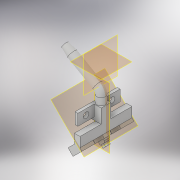
# Autodesk Inventor part: LickSensorMount_H
Saved by Autodesk Inventor 2020 (Build 240168000, 168)
## iProperties
Created: 2019-07-29
Part Number: LickSensorMount_H
Material: 일반
Document SubType Name: Modeling
Designer: Jeong Ji Hoon
Density: 1 g/cm^3
Appearance: 기본값
Author: Jeong Ji Hoon
## iProperties of the stored document _3D 인쇄.ipt
Created: 2020-01-15
Part Number: _3D 인쇄
Material: 일반
Document SubType Name: Modeling
Designer: Knowblesse
Density: 1 g/cm^3
Appearance: 기본값
Author: Knowblesse
Autodesk Inventor part; units mm, degrees
ref_plane "YZ Plane" through (0, 0, 0) normal (1, 0, 0) x (0, 1, 0)
ref_plane "XZ Plane" through (0, 0, 0) normal (0, 1, 0) x (-1, 0, 0)
ref_plane "XY Plane" through (0, 0, 0) normal (0, 0, 1) x (1, 0, 0)
sketch "스케치1" plane through (0, 0, 0) normal (0, 1, 0) x (-1, 0, 0)
  line L0 (0, 0) -> (7, 0)
  line L1 (7, 0) -> (7, -7)
  line L2 (7, -7) -> (0, -7)
  line L3 (0, -7) -> (0, 0)
  dimension "d0" = 7
  dimension "d1" = 7
  constraints: 8 end point, 2 parallel, 1 horizontal, 1 perpendicular
  measures "d0" distance of L1.end L2.end
  measures "d1" distance of L0.end L1.end
extrude "돌출1" add sketch "스케치1" along normal blind 10
sketch "스케치2" plane through (0, 10, 0) normal (0, 1, 0) x (1, 0, 0)
  line L0 (-7, 0) -> (0, 0) projected
  line L1 (0, 0) -> (0, 7) projected
  line L2 (0, 7) -> (-7, 7) projected
  line L3 (-7, 7) -> (-7, 0) projected
  circle A0 centre (-3.5, 3.5) radius 3
  line L4 (-7, 3.5) -> (0, 3.5) construction
  line L5 (-3.5, 7) -> (-3.5, 0) construction
  point P0 (-3.5, 3.5)
  dimension "d4" = 6
  constraints: 5 midpoint, 4 end point, 1 centre point, 1 coincident
  measures "d4" diameter of A0
extrude "돌출2" add sketch "스케치2" along normal blind 25 contours A0
ref_plane "작업 평면1" through (-3.5, 0, 0) normal (1, 0, 0) x (0, 0, -1)
sketch "스케치5" plane through (0, 0, 0) normal (1, 0, 0) x (0, 0, -1)
  line L0 (7, 0) -> (0, 0) projected
  line L1 (-15, -7) -> (22, -7)
  line L2 (22, -7) -> (22, 0)
  line L3 (22, 0) -> (-15, 0)
  line L4 (-15, 0) -> (-15, -7)
  point P0 (3.5, 0)
  dimension "d16" = 37
  dimension "d17" = 7
  constraints: 8 end point, 2 midpoint, 2 parallel, 1 horizontal, 1 perpendicular
  measures "d16" distance of L1.start L1.end
  measures "d17" distance of L3.end L1.start
extrude "돌출4" add sketch "스케치5" against normal blind 4
sketch "스케치6" plane through (0, 0, 0) normal (0, -1, 0) x (1, 0, 0)
  circle A0 centre (-3.5, -3.5) radius 2.5
  circle A1 centre (-3.5, -3.5) radius 3.5 projected
  dimension "d20" = 5
  constraints: 2 coincident, 1 centre point
  measures "d20" diameter of A0
extrude "돌출5" add sketch "스케치6" along normal blind 11 contours A0
ref_plane "작업 평면2" through (0, -7, 0) normal (0.7071068, 0.7071068, 0) x (0, 0, 1)
sketch "스케치7" plane through (0, -7, 0) normal (0.7071068, 0.7071068, 0) x (0, 0, 1)
  line L0 (-7, -4.9497) -> (-7, -12.0208) projected
  line L1 (0, -12.0208) -> (-7, -12.0208) projected
  line L2 (0, -4.9497) -> (0, -12.0208) projected
  line L3 (0, -4.9497) -> (15, -4.9497) projected
  line L4 (15, -4.9497) -> (15, 0) projected
  line L5 (15, 0) -> (-22, 0) projected
  line L6 (-22, 0) -> (-22, -4.9497) projected
  line L7 (-22, -4.9497) -> (-7, -4.9497) projected
  line L8 (-22, 2) -> (15, 2)
  line L9 (15, 2) -> (15, -3)
  line L10 (15, -3) -> (-22, -3)
  line L11 (-22, -3) -> (-22, 2)
  line L12 (15, -4.9497) -> (15, 0) projected
  dimension "d24" = 5
  dimension "d25" = 2
  constraints: 8 end point, 2 collinear, 2 parallel, 1 horizontal, 1 perpendicular
  measures "d24" distance of L8.end L9.end
  measures "d25" distance between parallel lines of L8 L5
extrude "돌출6" add sketch "스케치7" against normal blind 9 contours L6 L5 L4 L10 | L11 L8 L9 L5
sketch "스케치8" plane through (1.4142, -8.4142, 15) normal (0.7071068, -0.7071068, 0) x (-0.7071068, -0.7071068, 0)
  line L0 (0, 37) -> (0, 0) projected
  line L1 (0, 0) -> (9, 0) projected
  line L2 (9, 37) -> (9, 0) projected
  line L3 (0, 37) -> (9, 37) projected
  line L4 (0.9, 2.5) -> (7.2, 2.5)
  line L5 (7.2, 2.5) -> (7.2, 7.3)
  line L6 (7.2, 7.3) -> (0.9, 7.3)
  line L7 (0.9, 7.3) -> (0.9, 2.5)
  line L8 (0.9, 29.7) -> (7.2, 29.7)
  line L9 (7.2, 29.7) -> (7.2, 34.5)
  line L10 (7.2, 34.5) -> (0.9, 34.5)
  line L11 (0.9, 34.5) -> (0.9, 29.7)
  line L12 (9, 9.3) -> (0, 9.3)
  line L13 (9, 27.7) -> (0, 27.7)
  line L14 (9, 15.8) -> (0, 15.8)
  line L15 (9, 21.2) -> (0, 21.2)
  point P0 (-4.9497, 15)
  dimension "d28" = 6.3
  dimension "d29" = 4.8
  dimension "d31" = 2.5
  dimension "d32" = 1.8
  dimension "d33" = 2.5
  dimension "d34" = 2
  dimension "d35" = 2
  dimension "d36" = 6.5
  dimension "d37" = 6.5
  constraints: 24 end point, 10 point on line, 5 parallel, 5 perpendicular, 2 horizontal, 1 collinear
  measures "d28" distance of L5.end L6.end
  measures "d29" distance of L4.end L5.end
  measures "d31" distance between parallel lines of L1 L4
  measures "d32" distance between parallel lines of L2 L5
  measures "d33" distance between parallel lines of L3 L10
  measures "d34" distance between parallel lines of L6 L12
  measures "d35" distance between parallel lines of L8 L13
  measures "d36" distance between parallel lines of L12 L14
  measures "d37" distance between parallel lines of L13 L15
extrude "돌출7" cut sketch "스케치8" against normal through all contours L13 L2 L15 L0 | L14 L2 L12 L0 | L7 L6 L5 L4 | L11 L10 L9 L8
sketch "스케치9" plane through (1.4142, -8.4142, -0.8) normal (0.7071068, -0.7071068, 0) x (-0.7071068, -0.7071068, 0)
  line L0 (9, 5.4) -> (9, 0) projected
  line L1 (0, 5.4) -> (0, 0) projected
  line L2 (2, 0.7) -> (7, 0.7)
  line L3 (7, 0.7) -> (7, 4.7)
  line L4 (7, 4.7) -> (2, 4.7)
  line L5 (2, 4.7) -> (2, 0.7)
  line L6 (9, 2.7) -> (0, 2.7) construction
  point P0 (-4.9497, -0.8)
  point P1 (2, 2.7)
  dimension "d40" = 4
  dimension "d41" = 5
  dimension "d42" = 2
  constraints: 10 end point, 3 midpoint, 2 parallel, 1 horizontal, 1 perpendicular, 1 point on line
  measures "d40" distance of L2.end L3.end
  measures "d41" distance of L3.end L4.end
  measures "d42" distance between parallel lines of L3 L0
extrude "돌출8" add sketch "스케치9" along normal blind 2
sketch "스케치10" plane through (2.8284, -9.8284, -0.8) normal (0.7071068, -0.7071068, 0) x (0, 0, -1)
  line L0 (0.7, -2) -> (0.7, -7) projected
  line L1 (0.7, -7) -> (4.7, -7) projected
  line L2 (4.7, -7) -> (4.7, -2) projected
  line L3 (0.95, -4) -> (4.45, -4)
  line L4 (4.45, -4) -> (4.45, -6.5)
  line L5 (4.45, -6.5) -> (0.95, -6.5)
  line L6 (0.95, -6.5) -> (0.95, -4)
  point P0 (-0.8, 4.9497)
  dimension "d45" = 3.5
  dimension "d46" = 2.5
  dimension "d47" = 0.5
  dimension "d48" = 0.25
  dimension "d49" = 0.25
  constraints: 8 end point, 2 parallel, 1 horizontal, 1 perpendicular
  measures "d45" distance of L4.end L5.end
  measures "d46" distance of L3.end L4.end
  measures "d47" distance between parallel lines of L5 L1
  measures "d48" distance between parallel lines of L0 L6
  measures "d49" distance between parallel lines of L2 L4
extrude "돌출9" add sketch "스케치10" along normal blind 2
sketch "스케치11" plane through (4.2426, -11.2426, -0.8) normal (0.7071068, -0.7071068, 0) x (-0.7071068, -0.7071068, 0)
  line L0 (4, 4.45) -> (4, 0.95) projected
  line L1 (4, 0.95) -> (6.5, 0.95) projected
  line L2 (6.5, 0.95) -> (6.5, 4.45) projected
  line L3 (6.5, 4.45) -> (4, 4.45) projected
  line L4 (4.5, 1.45) -> (4.5, 3.95)
  line L5 (4.5, 3.95) -> (6, 3.95)
  line L6 (6, 3.95) -> (6, 1.45)
  line L7 (6, 1.45) -> (4.5, 1.45)
  point P0 (-4.9497, -0.8)
  dimension "d52" = 0.5
  constraints: 8 end point, 3 other
  measures "d52" distance between parallel lines of L0 L4
extrude "돌출10" cut sketch "스케치11" against normal blind 8 contours L4 L5 L6 L7
ref_plane "작업 평면3" through (-7, 10, -3.5) normal (0, 0, 1) x (1, 0, 0)
chamfer "모따기1" distance 1 angle 45 1 edges at (1.4142, -11.2426, -3.5)
sketch "스케치13" plane through (-4, -6.7574, 5.7) normal (0, 0, -1) x (-1, 0, 0)
  line L0 (0, 3.7574) -> (0, 0) projected
  line L1 (0, 0) -> (4.4853, -4.4853) projected
  line L2 (4.4853, -4.4853) -> (0.9497, -8.0208) projected
  line L3 (0.9497, -8.0208) -> (-5.4142, -1.6569) projected
  line L4 (-5.4142, -1.6569) -> (-4, -0.2426) projected
  line L5 (0, 3.7574) -> (-4, -0.2426) projected
  line L6 (0, 6.7574) -> (0, 3.7574) projected
  line L7 (-4, 6.7574) -> (0, 6.7574) projected
  line L8 (-4, -0.2426) -> (-4, 6.7574) projected
  line L9 (0, 0) -> (4.4853, -4.4853) projected
  line L10 (0, 3.7574) -> (0, 0) projected
  line L11 (0, 6.7574) -> (4.4853, -4.4853)
  point P0 (-1.1716, 1.1716)
  point P1 (0, 1.1716)
  constraints: 2 end point
extrude "돌출12" add sketch "스케치13" against normal up to surface (2 mm away) contours L6 L11 L1 L0
sketch "스케치14" plane through (-4, -6.7574, -12.7) normal (0, 0, 1) x (1, 0, 0)
  line L0 (-0.9497, -8.0208) -> (-4.4853, -4.4853) projected
  line L1 (-4.4853, -4.4853) -> (0, 0) projected
  line L2 (0, 0) -> (0, 3.7574) projected
  line L3 (4, -0.2426) -> (0, 3.7574) projected
  line L4 (4, -0.2426) -> (5.4142, -1.6569) projected
  line L5 (5.4142, -1.6569) -> (-0.9497, -8.0208) projected
  line L6 (0, 3.7574) -> (0, 6.7574) projected
  line L7 (0, 6.7574) -> (4, 6.7574) projected
  line L8 (4, 6.7574) -> (4, -0.2426) projected
  line L9 (0, 6.7574) -> (-4.4853, -4.4853)
  constraints: 2 end point
extrude "돌출13" add sketch "스케치14" against normal up to surface (2 mm away) contours L9 L6 L2 L1
ref_plane "작업 평면4" through (-3.5, 35, -3.5) normal (0, 1, 0) x (1, 0, 0)
sketch "스케치15" plane through (-3.5, 35, -3.5) normal (0, 1, 0) x (1, 0, 0)
  circle A0 centre (0, 0) radius 3.5 projected
  circle A1 centre (0, 0) radius 0.75
  point P0 (3.5, -3.5)
  dimension "d68" = 1.5
  constraints: 1 centre point, 1 coincident
  measures "d68" diameter of A1
extrude "돌출14" cut sketch "스케치15" against normal up to next contours A1
sketch "스케치16" plane through (-7, 0, 0) normal (-1, 0, 0) x (0, 0, 1)
  line L0 (0, 0) -> (-7, 0) projected
  line L1 (0, 0) -> (0, 10) projected
  line L2 (-7, 10) -> (0, 10) projected
  line L3 (-7, 0) -> (-7, 10) projected
  line L4 (11.5, 10) -> (-18.5, 10)
  line L5 (-18.5, 10) -> (-18.5, 2)
  line L6 (-18.5, 2) -> (11.5, 2)
  line L7 (11.5, 2) -> (11.5, 10)
  point P0 (-3.5, 10)
  dimension "d71" = 30
  dimension "d82" = 8
  constraints: 8 end point, 2 midpoint, 2 parallel, 1 collinear, 1 horizontal, 1 perpendicular
  measures "d71" distance of L5.end L6.end
  measures "d82" distance of L6.end L4.start
extrude "돌출15" add sketch "스케치16" against normal blind 2 contours L1 L4 L7 L6 | L6 L5 L4 L3
sketch "스케치17" plane through (-5, 0, 0) normal (1, 0, 0) x (0, 0, -1)
  line L0 (18.5, 2) -> (18.5, 10) projected
  line L1 (0, 0) -> (7, 0) projected
  line L2 (-11.5, 2) -> (-11.5, 10) projected
  line L3 (-11.5, 10) -> (18.5, 10) projected
  line L4 (18.5, 10) -> (18.5, 2) projected
  circle A0 centre (-5.75, 6) radius 2
  circle A1 centre (12.75, 6) radius 2
  line L5 (0, 0) -> (0, 2) projected
  line L6 (0, 2) -> (-11.5, 2) projected
  line L7 (18.5, 2) -> (7, 2) projected
  line L8 (7, 0) -> (7, 2) projected
  dimension "d74" = 4
  dimension "d75" = 4
  dimension "d76" = 5.75
  dimension "d77" = 5.75
  dimension "d81" = 4
  constraints: 2 centre point, 1 horizontal alignment
  measures "d74" diameter of A0
  measures "d75" diameter of A1
  measures "d76" distance from line of L0 A1.centre
  measures "d77" distance from line of L2 A0.centre
  measures "d81" distance from line of L3 A0.centre
extrude "돌출16" cut sketch "스케치17" against normal through all contours A0 | A1
sketch "스케치22" plane through (-3.5, 0, 0) normal (1, 0, 0) x (0, 0, -1)
  line L0 (6.5, 35) -> (0.5, 35) projected
  line L1 (0.5, 10) -> (6.5, 10) projected
  line L2 (0.5, 10) -> (0.5, 35) projected
  line L3 (2.75, 35) -> (4.25, 35) projected
  line L4 (3.5, 35) -> (3.5, 40)
  line L5 (6.5, 35) -> (0.5, 35) projected
  line L6 (0.5, 35) -> (0.5, 41)
  line L7 (0.5, 41) -> (1.3, 47)
  line L8 (1.3, 47) -> (2.1, 47)
  line L9 (2.1, 47) -> (2.1, 37)
  line L10 (2.1, 37) -> (2.75, 35)
  point P0 (0, 0)
  dimension "d113" = 5
  dimension "d114" = 10
  dimension "d115" = 2
  dimension "d116" = 0.8
  dimension "d117" = 6
  dimension "d118" = 2.8
  constraints: 12 end point, 2 perpendicular, 2 vertical, 1 midpoint
  measures "d113" distance of L4.start L4.end
  measures "d114" distance of L8.end L9.end
  measures "d115" distance from line of L9.end L0
  measures "d116" distance of L7.end L8.end
  measures "d117" vertical distance of L7.end L6.end
  measures "d118" diameter of L9 L4
revolve "회전4" add sketch "스케치22" angle 360 about axis through (-3.5, 35, -3.5) along (0, 1, 0)
sketch "스케치20" plane through (-3.5, 0, 0) normal (1, 0, 0) x (0, 0, -1)
  line L0 (6.5, 10) -> (6.5, 35) projected
  line L1 (0.5, 10) -> (0.5, 35) projected
  line L2 (6.5, 15) -> (0.5, 15)
  line L3 (0.5, 10) -> (6.5, 10) projected
  point P0 (0, 0)
  dimension "d86" = 5
  constraints: 2 end point, 2 point on line, 1 perpendicular
  measures "d86" distance between parallel lines of L2 L3
bend part "굽힘1" radius 5 angle 60 line through (-3.5, 15, -6.5) along (0, 0, 1) centre toward (-1, 0, 0) moving side (0, 1, 0) both sides no
